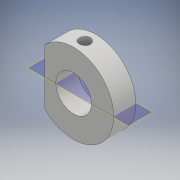
# Autodesk Inventor part: mocowanie uchwytu01
Saved by Autodesk Inventor 2017 (Build 210142000, 142)
## iProperties
Created: 2021-05-23
Part Number: mocowanie uchwytu01
Material: Generic
Document SubType Name: Modeling
Designer: majch
Density: 1 g/cm^3
Appearance: Default
Author: majch
Autodesk Inventor part; units mm, degrees
ref_plane "XZ Plane" through (0, 0, 0) normal (0, 1, 0) x (-1, 0, 0)
ref_plane "XY Plane" through (0, 0, 0) normal (0, 0, 1) x (1, 0, 0)
sketch "Sketch1" plane through (0, 0, 0) normal (0, 1, 0) x (-1, 0, 0)
  circle A0 centre (0, 0) radius 8
  arc A1 (12.9518, 12.5) -> (12.9518, -12.5) centre (0, 0) ccw
  line L0 (12.9518, 12.5) -> (12.9518, -12.5)
  dimension "d0" = 16
  dimension "d13" = 36
  dimension "d14" = 25
  constraints: 2 centre point, 2 coincident, 2 end point, 2 point on circle, 1 vertical
  measures "d0" diameter of A0
  measures "d13" diameter of A1
  measures "d14" distance of L0.start L0.end
extrude "Extrusion2" add sketch "Sketch1" along normal blind 10
sketch "Sketch3" plane through (-12.9518, 0, -12.5) normal (-1, 0, 0) x (0, 0, 1)
  circle A0 centre (21, 5) radius 2
  circle A1 centre (4, 5) radius 2
  line L0 (36, 5) -> (-7, 5) construction
  line L1 (25, 0) -> (0, 0) projected
  line L2 (25, 0) -> (25, 10) projected
  line L3 (0, 0) -> (0, 10) projected
  point P0 (12.5, 0)
  dimension "d17" = 4
  dimension "d18" = 4
  dimension "d19" = 5
  dimension "d20" = 17
  dimension "d21" = 4
  dimension "d22" = 25
  constraints: 2 centre point, 2 end point, 2 point on line
  measures "d17" diameter of A0
  measures "d18" diameter of A1
  measures "d19" distance between parallel lines of L0 L1
  measures "d20" distance of A1.centre A0.centre
  measures "d21" distance from line of L2 A0.centre
  measures "d22" distance between parallel lines of L2 L3
extrude "Extrusion3" cut sketch "Sketch3" against normal blind 6
ref_plane "Work Plane2" through (0, 0, 0) normal (0, 0, -1) x (0, 1, 0)
sketch "Sketch4" plane through (0, 0, 0) normal (0, 0, -1) x (0, 1, 0)
  circle A0 centre (5, 0) radius 2.5
  point P0 (0, 0)
  dimension "d26" = 5
  constraints: 1 centre point
  measures "d26" diameter of A0
hole "Hole1" at (0, 5, 0) direction (0, 0, 1) diameter 5 end through all
equation "\"d21\" = -0.5 * d20 + 0.5 * d22"
body "Solid2"
